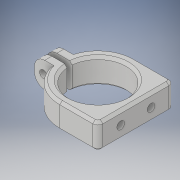
# Autodesk Inventor part: ScreenMount
Saved by Autodesk Inventor 2019.3 (Build 233278000, 278)
## iProperties
Created: 2019-04-04
Part Number: ScreenMount
Material: Типовые
Document SubType Name: Modeling
Designer: Andrew
Density: 1 g/cm^3
Appearance: По умолчанию
Author: Andrew
Autodesk Inventor part; units mm, degrees
ref_plane "YZ Plane" through (0, 0, 0) normal (1, 0, 0) x (0, 1, 0)
ref_plane "XZ Plane" through (0, 0, 0) normal (0, 1, 0) x (-1, 0, 0)
ref_plane "XY Plane" through (0, 0, 0) normal (0, 0, 1) x (1, 0, 0)
sketch "Эскиз1" plane through (0, 0, 0) normal (0, 1, 0) x (-1, 0, 0)
  arc A0 (11.1553, 1) -> (11.1553, -1) centre (0, 0) ccw
  line L0 (-15, 15) -> (-15, -15)
  line L1 (-15, 15) -> (0, 15)
  line L2 (-15, -15) -> (0, -15)
  line L3 (11.1553, 1) -> (14.9666, 1)
  line L4 (14.9666, -1) -> (11.1553, -1)
  arc A1 (0, -15) -> (14.5107, -3.8) centre (0, 0) ccw
  arc A2 (14.5107, 3.8) -> (0, 15) centre (0, 0) ccw
  line L5 (11.1553, -1) -> (21.1553, -1)
  line L6 (21.1553, -1) -> (21.1553, -3.8)
  line L7 (21.1553, -3.8) -> (14.5107, -3.8)
  line L8 (11.1553, 1) -> (21.1553, 1)
  line L9 (21.1553, 1) -> (21.1553, 3.8)
  line L10 (21.1553, 3.8) -> (14.5107, 3.8)
  point P0 (15, 0)
  dimension "d0" = 22.4
  dimension "d2" = 30
  dimension "d5" = 2.8
  dimension "d6" = 2.8
  constraints: 22 end point, 6 point on circle, 4 parallel, 3 centre point, 3 horizontal, 2 coincident, 2 perpendicular, 2 tangent, 1 vertical
  measures "d0" diameter of A0
  measures "d2" distance of L0.start L0.end
  measures "d5" distance between parallel lines of L7 L5
  measures "d6" distance of L8.end L9.end
extrude "Выдавливание1" add sketch "Эскиз1" along normal blind 10
sketch "Эскиз2" plane through (15, 0, 15) normal (1, 0, 0) x (0, 0, -1)
  line L0 (0, 0) -> (30, 0) projected
  line L1 (30, 0) -> (30, 10) projected
  line L2 (0, 10) -> (30, 10) projected
  line L3 (0, 0) -> (0, 10) projected
  line L4 (0, 5) -> (30, 5) construction
  line L5 (15, 10) -> (15, 0) construction
  point P0 (21, 5)
  point P1 (9, 5)
  dimension "d10" = 6
  dimension "d11" = 6
  constraints: 4 end point, 3 midpoint, 2 point on line, 1 vertical
  measures "d10" distance from line of L5 point (21, 5)
  measures "d11" distance from line of L5 point (9, 5)
hole "Отверстие1" at (15, 5, -6) at (15, 5, 6) direction (-1, 0, 0) diameter 3 depth 8 tip angle 118
fillet "Сопряжение1" radius 4 4 edges at (-21.1553, 10, 2.4) (-21.1553, 10, -2.4) (-21.1553, 0, 2.4) (-21.1553, 0, -2.4)
sketch "Эскиз3" plane through (-14.5107, 0, 3.8) normal (0, 0, 1) x (1, 0, 0)
  arc A0 (-6.6446, 4) -> (-2.6446, 0) centre (-2.6446, 4) ccw projected
  line L0 (-2.6446, 0) -> (0, 0) projected
  line L1 (0, 0) -> (0, 10) projected
  line L2 (-2.6446, 10) -> (0, 10) projected
  arc A1 (-2.6446, 10) -> (-6.6446, 6) centre (-2.6446, 6) ccw projected
  line L3 (-6.6446, 4) -> (-6.6446, 6) projected
  line L4 (-6.6446, 5) -> (-3.1446, 5) construction
  point P0 (14.5107, 0)
  dimension "d20" = 3.5
  constraints: 2 end point, 1 coincident, 1 horizontal, 1 midpoint
  measures "d20" distance of L4.start L4.end
hole "Отверстие2" at (-17.6553, 5, 3.8) direction (0, 0, -1) diameter 3 depth 8 tip angle 118
fillet "Сопряжение2" radius 2 2 edges at (15, 5, 15) (15, 5, -15)
chamfer "Фаска1" distance 1 angle 45 16 edges at (11.2, 10, 0) (11.2, 0, 0) (6.5, 10, 15) (14.4142, 10, 14.4142) (15, 10, 0) (14.4142, 10, -14.4142) (6.5, 10, -15) (-9.1652, 10, -11.8743) (-9.1652, 10, 11.8743) (6.5, 0, 15) (14.4142, 0, 14.4142) (15, 0, 0) (14.4142, 0, -14.4142) (6.5, 0, -15) (-9.1652, 0, -11.8743) (-9.1652, 0, 11.8743)
